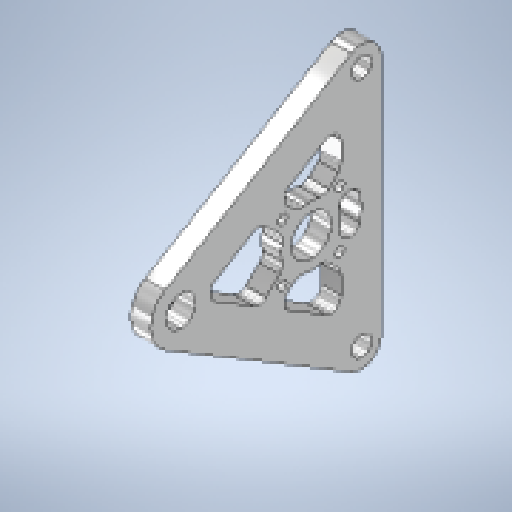
# Autodesk Inventor part: Frame (Motor Side)
Saved by Autodesk Inventor 2023 (Build 270158000, 158)
## iProperties
Created: 2022-05-22
Part Number: Frame (Motor Side)
Material: Aluminum 6061
Document SubType Name: Modeling
Designer: Nathan Cai
Density: 2.7 g/cm^3
Appearance: Aluminum - Flat
Mass: 51.1911 g
Surface Area: 97.1122 cm^2
Volume: 18.9597 cm^3
Author: Nathan Cai
Autodesk Inventor part; units mm, degrees
ref_plane "YZ Plane" through (0, 0, 0) normal (1, 0, 0) x (0, 1, 0)
ref_plane "XZ Plane" through (0, 0, 0) normal (0, 1, 0) x (-1, 0, 0)
ref_plane "XY Plane" through (0, 0, 0) normal (0, 0, 1) x (1, 0, 0)
sketch "Sketch1" plane through (0, 0, 0) normal (1, 0, 0) x (0, 1, 0)
  circle A0 centre (0, 0) radius 6.35
  circle A1 centre (0, 0) radius 22.225
  line L0 (0, 0) -> (0, 41.275) construction
  circle A2 centre (0, 41.275) radius 4.7625
  circle A3 centre (0, 41.275) radius 76.2 construction
  circle A4 centre (0, 41.275) radius 9.525
  line L1 (0, -15.875) -> (38.1, -15.875) construction
  circle A5 centre (38.1, -15.875) radius 3.175
  arc A6 (32.6593, -19.1494) -> (43.5407, -12.6006) centre (38.1, -15.875) ccw
  line L2 (8.161, 46.1865) -> (43.5407, -12.6006)
  line L3 (1.9103, 31.9435) -> (32.6593, -19.1494)
  circle A7 centre (-38.1, -15.875) radius 3.175
  arc A8 (-43.5407, -12.6006) -> (-32.6593, -19.1494) centre (-38.1, -15.875) ccw
  line L4 (-8.161, 46.1865) -> (-43.5407, -12.6006)
  line L5 (-1.9103, 31.9435) -> (-32.6593, -19.1494)
  line L6 (0, 0) -> (0, -9.5) construction
  line L7 (0, 0) -> (9.5, 0) construction
  line L8 (0, 0) -> (-8, 0) construction
  line L9 (0, 0) -> (-12.5, 0) construction
  line L10 (0, 0) -> (12.7, 0) construction
  line L11 (0, 0) -> (4.3437, -11.9341) construction
  line L12 (38.1, -15.875) -> (7.351, 35.2179) construction
  line L13 (-9, 9) -> (9, 9) construction
  line L14 (9, 9) -> (9, -9) construction
  line L15 (9, -9) -> (-9, -9) construction
  line L16 (-9, -9) -> (-9, 9) construction
  line L17 (-9, 9) -> (9, -9) construction
  line L18 (9, 9) -> (-9, -9) construction
  line L19 (-9, 9) -> (9, 9) construction
  circle A9 centre (9, -9) radius 1.5
  circle A10 centre (9, 9) radius 1.5
  circle A11 centre (-9, 9) radius 1.5
  circle A12 centre (-9, -9) radius 1.5
  arc A13 (3.287, 12.2673) -> (-3.287, 12.2673) centre (0, 0) ccw construction
  arc A14 (4.1088, 15.3341) -> (-4.1088, 15.3341) centre (0, 0) ccw
  arc A15 (2.4653, 9.2004) -> (-2.4653, 9.2004) centre (0, 0) ccw
  arc A16 (2.4653, 9.2004) -> (4.1088, 15.3341) centre (3.287, 12.2673) ccw
  arc A17 (-4.1088, 15.3341) -> (-2.4653, 9.2004) centre (-3.287, 12.2673) ccw
  line L20 (0, 0) -> (-3.287, 12.2673) construction
  line L21 (0, 0) -> (3.287, 12.2673) construction
  arc A18 (-9.2004, 2.4653) -> (-9.2004, -2.4653) centre (0, 0) ccw
  arc A19 (-9.2004, 2.4653) -> (-15.3341, 4.1088) centre (-12.2673, 3.287) ccw
  arc A20 (-15.3341, -4.1088) -> (-9.2004, -2.4653) centre (-12.2673, -3.287) ccw
  arc A21 (-12.2673, 3.287) -> (-12.2673, -3.287) centre (0, 0) ccw construction
  arc A22 (-15.3341, 4.1088) -> (-15.3341, -4.1088) centre (0, 0) ccw
  arc A23 (-2.4653, -9.2004) -> (2.4653, -9.2004) centre (0, 0) ccw
  arc A24 (-2.4653, -9.2004) -> (-4.1088, -15.3341) centre (-3.287, -12.2673) ccw
  arc A25 (4.1088, -15.3341) -> (2.4653, -9.2004) centre (3.287, -12.2673) ccw
  arc A26 (-3.287, -12.2673) -> (3.287, -12.2673) centre (0, 0) ccw construction
  arc A27 (-4.1088, -15.3341) -> (4.1088, -15.3341) centre (0, 0) ccw
  arc A28 (9.2004, -2.4653) -> (9.2004, 2.4653) centre (0, 0) ccw
  arc A29 (9.2004, -2.4653) -> (15.3341, -4.1088) centre (12.2673, -3.287) ccw
  arc A30 (15.3341, 4.1088) -> (9.2004, 2.4653) centre (12.2673, 3.287) ccw
  arc A31 (12.2673, -3.287) -> (12.2673, 3.287) centre (0, 0) ccw construction
  arc A32 (15.3341, -4.1088) -> (15.3341, 4.1088) centre (0, 0) ccw
  line L22 (38.1, -22.225) -> (-38.1, -22.225)
  line L23 (26.8671, -9.525) -> (-26.8671, -9.525)
  line L24 (-11.5072, 15.9973) -> (-5.5321, 10.0222)
  line L25 (11.5072, 15.9973) -> (5.5321, 10.0222)
  line L26 (14.8811, 10.391) -> (10.0222, 5.5321)
  line L27 (-14.8811, 10.391) -> (-10.0222, 5.5321)
  line L28 (-10.0222, -5.5321) -> (-14.0151, -9.525)
  line L29 (10.0222, -5.5321) -> (14.0151, -9.525)
  point P0 (9.2604, -20.2038)
  point P1 (-1.9103, 31.9435)
  point P2 (19.107, 3.3693)
  point P3 (-11.4476, -19.05)
  point P4 (-20.0805, -9.525)
  point P5 (20.0805, -9.525)
  point P6 (0, -22.225)
  point P7 (5.5321, 10.0222)
  point P8 (-10.0222, 5.5321)
  point P9 (-13.1031, -6.35)
  point P10 (13.1031, -6.35)
  point P11 (12.0702, 18.6618)
  point P12 (0, 22.225)
  point P13 (-12.0702, 18.6618)
  point P14 (-11.6515, -6.4017)
  point P15 (9.9271, 7.8208)
  point P16 (10.306, 9.7378)
  point P17 (-10.306, 9.7378)
  point P18 (-9.9271, 7.8208)
  point P19 (8.8708, 20.3779)
  point P20 (22.1597, -1.703)
  point P21 (-22.1597, -1.703)
  point P22 (-8.8708, 20.3779)
  dimension "d1" = 44.45
  dimension "d0" = 12.7
  dimension "d3" = 9.525
  dimension "d4" = 152.4
  dimension "d5" = 19.05
  dimension "d6" = 38.1
  dimension "d7" = 6.35
  dimension "d8" = 12.7
  dimension "d10" = 12.7
  dimension "d15" = 9.5
  dimension "d16" = 270
  dimension "d18" = 8
  dimension "d20" = 12.5
  dimension "d35" = 70
  dimension "d38" = 18
  dimension "d40" = 18
  dimension "d41" = 3
  dimension "d44" = 360
  dimension "d46" = 12.7
  dimension "d47" = 30
  dimension "d48" = 6.35
  dimension "d49" = 75
  dimension "d52" = 360
  dimension "d58" = 15.875
  dimension "d59" = 57.15
  constraints: 60 end point, 53 point on circle, 32 centre point, 13 tangent, 12 coincident, 12 symmetric about line, 8 parallel, 8 point on line, 4 horizontal, 3 midpoint, 2 equal length, 2 perpendicular, 1 collinear, 1 vertical, 64 other
  measures "d0" diameter of A0
  measures "d3" diameter of A2
  measures "d4" diameter of A3
  measures "d5" diameter of A4
  measures "d6" distance of L1.start L1.end
  measures "d7" diameter of A5
  measures "d8" diameter of A6
  measures "d10" distance between parallel lines of L2 L3
  measures "d15" distance of L0.start L6.end
  measures "d18" distance of L0.start L8.end
  measures "d20" distance of L0.start L9.end
  measures "d35" angle of L7 L11
  measures "d38" distance of L13.start L13.end
  measures "d40" distance of L13.end L14.end
  measures "d41" diameter of A9
  measures "d46" radius of A13
  measures "d47" angle of L21 L20
  measures "d48" diameter of A17
  measures "d49" angle of L7 L21
  measures "d58" distance from line of point (0, 0) L1
  measures "d59" distance from line of A2.centre L1
extrude "Extrusion1" add sketch "Sketch1" along normal blind 6.35 contours A1 L3 | A1 L3 A4 L2 A6 | L5 A1 | A1 L5 A8 L4 A4 | A4 | L3 L26 A30 A28 A29 L29 L23 A9 A25 A23 A24 A12 L28 A20 A18 A19 L27 L5 L24 A17 A15 A16 L25 | L23 L3 A6 L22 A1 | A1 L23 A12 A24 A27 A25 A9 | L22 A8 L5 L23 A1
fillet "Fillet2" radius 3.175 10 edges at (3.175, 1.9103, 31.9435) (3.175, -1.9103, 31.9435) (3.175, 14.8811, 10.391) (3.175, 11.5072, 15.9973) (3.175, 26.8671, -9.525) (3.175, 14.0151, -9.525) (3.175, -14.0151, -9.525) (3.175, -26.8671, -9.525) (3.175, -14.8811, 10.391) (3.175, -11.5072, 15.9973)
equation "\"d10\" = d8"
body "Solid1"
